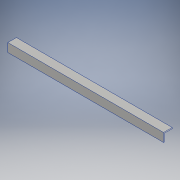
# Autodesk Inventor part: SUP_006_FlywheelLBracketMount
Saved by Autodesk Inventor 2018.3 (Build 223284000, 284)
## iProperties
Created: 2020-01-31
Part Number: SUP_006_FlywheelLBracketMount
Material: Aluminum 6061
Document SubType Name: Modeling
Designer: 21hickjosh
Density: 2.7 g/cm^3
Appearance: Aluminum - Flat
Mass: 186.659 g
Surface Area: 467.539 cm^2
Volume: 69.1329 cm^3
Author: 21hickjosh
Autodesk Inventor part; units mm, degrees
ref_plane "YZ Plane" through (0, 0, 0) normal (1, 0, 0) x (0, 1, 0)
ref_plane "XZ Plane" through (0, 0, 0) normal (0, 1, 0) x (-1, 0, 0)
ref_plane "XY Plane" through (0, 0, 0) normal (0, 0, 1) x (1, 0, 0)
sketch "Sketch1" plane through (0, 0, 0) normal (0, 0, 1) x (1, 0, 0)
  line L0 (0, 0) -> (0, 25.4)
  line L1 (0, 25.4) -> (3.175, 25.4)
  line L2 (0, 0) -> (25.4, 0)
  line L3 (25.4, 0) -> (25.4, 3.175)
  line L4 (25.4, 3.175) -> (3.175, 3.175)
  line L5 (3.175, 3.175) -> (3.175, 25.4)
  dimension "d0" = 25.4
  dimension "d1" = 3.175
  dimension "d2" = 25.4
  dimension "d3" = 3.175
  constraints: 12 end point, 4 perpendicular, 1 horizontal, 1 vertical
  measures "d0" distance of L0.start L0.end
  measures "d1" distance of L0.end L1.end
  measures "d2" distance of L0.start L2.end
  measures "d3" distance of L2.end L3.end
extrude "Extrusion1" add sketch "Sketch1" along normal blind 457.2
body "Solid1"
